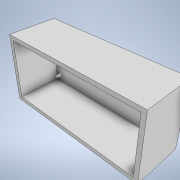
# Autodesk Inventor part: laatikko
Saved by Autodesk Inventor 2020.1 (Build 241239000, 239)
## iProperties
Created: 2021-11-03
Part Number: laatikko
Material: Generic
Document SubType Name: Modeling
Designer: s1mate03
Density: 1 g/cm^3
Appearance: Default
Author: s1mate03
Autodesk Inventor part; units mm, degrees
ref_plane "YZ Plane" through (0, 0, 0) normal (1, 0, 0) x (0, 1, 0)
ref_plane "XZ Plane" through (0, 0, 0) normal (0, 1, 0) x (-1, 0, 0)
ref_plane "XY Plane" through (0, 0, 0) normal (0, 0, 1) x (1, 0, 0)
sketch "Sketch1" plane through (0, 0, 0) normal (0, 0, 1) x (1, 0, 0)
  line L0 (0, 0) -> (68, 0)
  line L1 (68, 0) -> (68, -32)
  line L2 (68, -32) -> (0, -32)
  line L3 (0, -32) -> (0, 0)
  dimension "d0" = 68
  dimension "d1" = 32
  constraints: 8 end point, 2 parallel, 1 horizontal, 1 perpendicular
  measures "d0" distance of L0.start L0.end
  measures "d1" distance of L2.end L0.start
extrude "Extrusion1" add sketch "Sketch1" along normal blind 23
shell "Shell1" thickness 2 removed faces 1 at (22.6667, -10.6667, 23)
sketch "Sketch5" plane through (2, -30, 2) normal (0, 0, 1) x (1, 0, 0)
  line L0 (-2, 30) -> (3, 30)
  line L1 (66, 30) -> (-2, 30) projected
  line L2 (3, 30) -> (3, 14)
  line L3 (3, 14) -> (3, 24.25)
  line L4 (3, 24.25) -> (60.5, 24.25)
  line L5 (60.5, 24.25) -> (60.5, 3.75)
  line L6 (60.5, 3.75) -> (3, 3.75)
  line L7 (3, 3.75) -> (3, 14)
  circle A0 centre (60.5, 24.25) radius 0.75
  circle A1 centre (60.5, 3.75) radius 0.75
  circle A2 centre (3, 24.25) radius 0.75
  circle A3 centre (3, 3.75) radius 0.75
  dimension "d5" = 5
  dimension "d6" = 16
  dimension "d7" = 10.25
  dimension "d8" = 57.5
  dimension "d9" = 20.5
  dimension "d10" = 1.5
  dimension "d11" = 1.5
  dimension "d12" = 1.5
  dimension "d13" = 1.5
  constraints: 14 end point, 5 perpendicular, 4 centre point, 4 coincident, 3 point on line
  measures "d5" distance of L0.start L0.end
  measures "d6" distance of L0.end L2.end
  measures "d7" distance of L2.end L3.end
  measures "d8" distance of L3.end L4.end
  measures "d9" distance of L4.end L5.end
  measures "d10" diameter of A0
  measures "d11" diameter of A1
  measures "d12" diameter of A2
  measures "d13" diameter of A3
extrude "Extrusion2" add sketch "Sketch5" along normal blind 3 contours A2 L4 L2 | L2 A2 | L4 A2 L2 | A0 L5 L4 | L4 L5 A0 | A3 L6 L7 | L7 L6 A3 | A1 L6 L5 | L5 L6 A1
body "Solid1"
